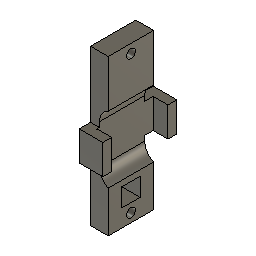
gearbox_bracket (Autodesk Fusion 360 design; units mm, degrees)
Autodesk Fusion 360 part; units mm, degrees
sketch "Sketch1" plane through (0, 0, 0) normal (0, 0, 1) x (1, 0, 0) in component "front bracket"
  line L0 (0, 0) -> (15.326, 0)
  line L1 (15.326, 0) -> (15.326, 42.5)
  line L2 (15.326, 42.5) -> (0, 42.5)
  line L3 (0, 42.5) -> (0, 0)
  line L4 (0, 0) -> (15.326, 0)
  line L5 (15.326, 0) -> (15.326, 10)
  line L6 (15.326, 10) -> (0, 10)
  line L7 (0, 10) -> (0, 0)
  line L8 (0, 42.5) -> (15.326, 42.5)
  line L9 (15.326, 42.5) -> (15.326, 32.5)
  line L10 (15.326, 32.5) -> (0, 32.5)
  line L11 (0, 32.5) -> (0, 42.5)
  circle A0 centre (7.663, 37) radius 1.35
  line L12 (10.763, 8.1) -> (4.563, 8.1)
  line L13 (4.563, 8.1) -> (4.563, 1.9)
  line L14 (4.563, 1.9) -> (10.763, 1.9)
  line L15 (10.763, 1.9) -> (10.763, 8.1)
  line L16 (10.763, 8.1) -> (4.563, 1.9) construction
  line L17 (4.563, 8.1) -> (10.763, 1.9) construction
  line L18 (15.326, 32.5) -> (18.163, 32.5)
  line L19 (0, 32.5) -> (-0.837, 32.5)
  line L20 (15.326, 10) -> (18.163, 10)
  line L21 (0, 10) -> (-0.837, 10)
  line L22 (-0.837, 32.5) -> (-0.837, 10)
  line L23 (18.163, 32.5) -> (18.163, 10)
  line L24 (18.163, 21.25) -> (21.163, 21.25)
  line L25 (21.163, 21.25) -> (21.163, 26.25)
  line L26 (21.163, 26.25) -> (18.163, 26.25)
  line L27 (18.163, 26.25) -> (18.163, 21.25)
  line L28 (-0.837, 21.25) -> (-3.837, 21.25)
  line L29 (-3.837, 21.25) -> (-3.837, 26.25)
  line L30 (-3.837, 26.25) -> (-0.837, 26.25)
  line L31 (-0.837, 26.25) -> (-0.837, 21.25)
  line L32 (-3.837, 21.25) -> (-3.837, 16.25)
  line L33 (-3.837, 16.25) -> (-0.837, 16.25)
  line L34 (21.163, 16.25) -> (18.163, 16.25)
  line L35 (21.163, 21.25) -> (21.163, 16.25)
  line L36 (-0.837, 26.25) -> (0, 26.25)
  line L37 (-0.837, 16.25) -> (0, 16.25)
  line L38 (18.163, 26.25) -> (15.326, 26.25)
  line L39 (18.163, 16.25) -> (15.326, 16.25)
  circle A1 centre (7.663, 37) radius 2.5
  point P0 (7.663, 5)
  dimension "d1" = 15.326
  dimension "d2" = 42.5
  dimension "d3" = 10
  dimension "d4" = 10
  dimension "d5" = 2.7
  dimension "d6" = 4.5
  dimension "d7" = 7.663
  dimension "d8" = 6.2
  dimension "d9" = 6.2
  dimension "d10" = 1.9
  dimension "d11" = 4.563
  dimension "d12" = 2.837
  dimension "d13" = 0.837
  dimension "d14" = 2.837
  dimension "d15" = 0.837
  dimension "d16" = 3
  dimension "d17" = 5
  dimension "d18" = 3
  dimension "d19" = 5
  dimension "d30" = 5
  constraint horizontal L0
  constraint vertical L1
  constraint horizontal L2
  constraint vertical L3
  constraint coincident L0.start L3.end
  constraint horizontal L4
  constraint vertical L5
  constraint horizontal L6
  constraint vertical L7
  constraint horizontal L8
  constraint vertical L9
  constraint horizontal L10
  constraint vertical L11
  constraint coincident L1 L9.end
  constraint horizontal L12
  constraint perpendicular L12 L13
  constraint parallel L12 L14
  constraint parallel L13 L15
  constraint coincident L16 P0
  constraint coincident L17 P0
  constraint perpendicular L9 L18
  constraint perpendicular L11 L19
  constraint perpendicular L1 L20
  constraint perpendicular L3 L21
  constraint perpendicular L20 L23
  constraint horizontal L24
  constraint vertical L25
  constraint horizontal L26
  constraint vertical L27
  constraint midpoint L23 L24.start
  constraint horizontal L28
  constraint vertical L29
  constraint horizontal L30
  constraint vertical L31
  constraint midpoint L22 L28.start
  constraint symmetric L25.start L24 L35.start
  constraint symmetric L25.end L24 L34.start
  constraint symmetric L26.end L24 L34.end
  constraint symmetric L24 L28.end L29.start
  constraint symmetric L24 L29.end L32.end
  constraint symmetric L24 L30.end L33.end
  constraint coincident L3 L36.end
  constraint perpendicular L3 L36
  constraint coincident L3 L37.end
  constraint perpendicular L3 L37
  constraint coincident L1 L38.end
  constraint perpendicular L1 L38
  constraint coincident L1 L39.end
  constraint perpendicular L1 L39
  constraint concentric A0 A1
  measures "d1" distance of L0.start L0.end
  measures "d2" distance of L0.start L2.end
  measures "d3" distance of L0.start L6.end
  measures "d4" distance of L2.end L10.end
  measures "d5" diameter of A0
  measures "d6" distance of L10 A0.centre
  measures "d7" distance of L11 A0.centre
  measures "d8" distance of L13.end L14.end
  measures "d9" distance of L12.end L13.end
  measures "d10" distance of L4 L14
  measures "d11" distance of L1 L15
  measures "d12" distance of L9.end L18.end
  measures "d13" distance of L10.end L19.end
  measures "d14" distance of L5.end L20.end
  measures "d15" distance of L6.end L21.end
  measures "d16" distance of L24.start L24.end
  measures "d17" distance of L24.start L26.end
  measures "d18" distance of L28.start L28.end
  measures "d19" distance of L28.start L30.end
  measures "d30" diameter of A1
extrude "Extrude1" add sketch "Sketch1" along normal blind 5 contours L0 L1 L3 L4 L5 L6 L7 | L22 L28 L32 L33 | L23 L24 L34 L35 | L1 L2 L3 L8 L9 L10 L11 | L22 L28 L29 L30 L31 | L23 L24 L25 L26 L27 | A1 makes body 1 at (-0.837, 22.9167, 1.6667) makes body 2 at (18.163, 22.9167, 1.6667) makes body 3 at (2.1094, 37.4004, 0) makes body 4 at (13.805, 3.9667, 0) in component "front bracket"
extrude "Extrude2" add sketch "Sketch1" against normal blind 3 contours L0 L1 L3 L4 L5 L6 L7 | L1 L3 L6 L10 | L3 L22 L31 L36 L37 | L1 L23 L27 L38 L39 | L22 L28 L32 L33 | L23 L24 L34 L35 | L1 L2 L3 L8 L9 L10 L11 | L22 L28 L29 L30 L31 | L23 L24 L25 L26 L27 | A1 bodies 1 2 3 4 in component "front bracket"
extrude "Extrude3" cut 2 faces at (2.1094, 37.4004, 5) (13.805, 3.9667, 5) along direction (0, 0, -1) blind 2 on bodies 1 bodies 1 in component "front bracket"
fillet "Fillet2" radius 5 2 edges at (7.663, 10, 0) (7.663, 32.5, 0) on bodies 1 in component "front bracket"
extrude "Extrude4" cut sketch "Sketch1" against normal blind 3 contours A1 bodies 1 in component "front bracket"
extrude "Extrude5" add 1 faces at (9.7653, 36.8087, 0) along direction (0, 0, -1) blind 1 on bodies 1 bodies 1 in component "front bracket"
move_face "OffsetFaces1" offset 4 1 faces at (5.1087, 0, 1) on bodies 1 in component "front bracket"
sketch "Sketch1 (2)" plane through (0.0367, 0.1136, 3) normal (0, 0, 1) x (-1, 0, 0)
  line L0 (-10.7263, -7.9864) -> (-10.7263, -1.7864)
  line L1 (-10.7263, -1.7864) -> (-4.5263, -1.7864)
  line L2 (-4.5263, -1.7864) -> (-4.5263, -7.9864)
  line L3 (-4.5263, -7.9864) -> (-10.7263, -7.9864)
  line L4 (0.0367, -9.8864) -> (0.0367, 4.1136)
  line L5 (0.0367, 4.1136) -> (-15.2893, 4.1136)
  line L6 (-15.2893, 4.1136) -> (-15.2893, -9.8864)
  line L7 (-15.2893, -9.8864) -> (0.0367, -9.8864)
  circle A0 centre (-7.6263, 1.1636) radius 1.5
  dimension "d36" = 3
  measures "d36" diameter of A0
hole "Hole1" at (7.663, -1.05, 3) direction (0, 0, -1) diameter 3 depth 6 tip angle 180 bodies 1 in component "front bracket"
extrude "Extrude6" add 1 faces at (5.1087, 42.5, -1) along direction (0, 1, 0) blind 6 on bodies 1 bodies 1 in component "front bracket"
sketch "Sketch2" plane through (0, 0, 3) normal (0, 0, 1) x (-1, 0, 0)
  circle A0 centre (-7.663, -37) radius 1.35
  line L0 (0, -32.5) -> (-15.326, -32.5)
  line L1 (-15.326, -32.5) -> (-15.326, -48.5)
  line L2 (-15.326, -48.5) -> (0, -48.5)
  line L3 (0, -48.5) -> (0, -32.5)
  line L4 (-7.663, -48.5) -> (-7.663, -42.5)
  circle A1 centre (-7.663, -45.5) radius 1.5
  dimension "d42" = 6
  dimension "d43" = 3
  constraint midpoint L2 L4.start
  constraint perpendicular L2 L4
  constraint midpoint L4 A1.centre
  measures "d42" distance of L4.start L4.end
  measures "d43" diameter of A1
hole "Hole2" at (7.663, 45.5, 3) direction (0, 0, -1) diameter 2.7 depth 6 tip angle 180 bodies 1 in component "front bracket"
delete_face "DeleteFace1" 1 faces at (6.3197, 36.8656, 0.3333) on bodies 1 in component "front bracket"
extrude "Extrude7" add 1 faces at (8.4138, 36.6384, -1) along direction (0, 0, -1) blind 2 on bodies 1 bodies 1 in component "front bracket"
move_face "OffsetFaces2" offset -0.15 1 faces at (7.7303, 44.1517, 1) on bodies 1 in component "front bracket"
move_body "Move1" bodies 1 to x (0, 1, 0) y (-1, 0, 0) z (0, 0, 1) at (0, 0, 0) in component "front bracket"
move_body "Move2" bodies 1 to x (1, 0, 0) y (0, 1, 0) z (0, 0, 1) at (21.5943, -8.1971, -0.2355) in component "front bracket"
move_body "Move3" bodies 1 to x (0, 0, -1) y (0, 1, 0) z (1, 0, 0) at (0.5798, 0, 0.1087) in component "front bracket"
move_body "Move4" bodies 1 to x (1, 0, 0) y (0, 1, 0) z (0, 0, 1) at (0, 1, 13.15) in component "front bracket"
move_body "Move5" bodies 1 to x (1, 0, 0) y (0, 1, 0) z (0, 0, 1) at (0, 0, 3.1) in component "front bracket"
component "front bracket" placed x (1, 0, 0) y (0, 1, 0) z (0, 0, 1) at (-0.3443, -0.4659, 0.2355)
equation "d49 = ( -0.3 / 2 ) * 1 mm"
